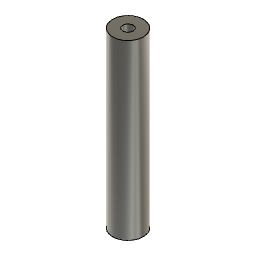
Leg_Link_1 v1 (Autodesk Fusion 360 design; units mm, degrees)
Autodesk Fusion 360 part; units mm, degrees
sketch "Sketch1" plane through (0, 0, 0) normal (0, 0, 1) x (1, 0, 0)
  circle A0 centre (0, 0) radius 4.5
  circle A1 centre (0, 0) radius 1.5
  dimension "d1" = 9
  dimension "d2" = 3
  constraint coincident A0.centre A1.centre
  constraint concentric A0 A1
  measures "d1" diameter of A0
  measures "d2" diameter of A1
extrude "Extrude1" add sketch "Sketch1" against normal blind 50.8 contours A0 | A1
extrude "Extrude2" cut sketch "Sketch1" against normal blind 10 contours A1
sketch "Sketch2" plane through (0, 0, -50.8) normal (0, 0, -1) x (1, 0, 0)
  circle A0 centre (0, 0) radius 4.5
  circle A1 centre (0, 0) radius 1.5
extrude "Extrude3" cut sketch "Sketch2" against normal blind 10 contours A1
equation "d3 = -25.4 * 2 mm"
